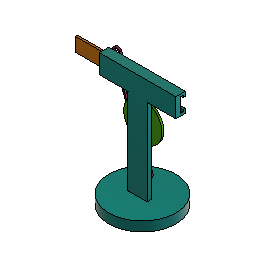
Crank-and-slotted-link-mechanism (Autodesk Fusion 360 design; units mm, degrees)
Autodesk Fusion 360 part; units mm, degrees
sketch "Base" plane through (0, 0, 0) normal (0, 1, 0) x (1, 0, 0) in component "Holder Base"
  circle A0 centre (0, 0) radius 35
  dimension "d1" = 70
  constraint coincident A0.centre origin
  measures "d1" diameter of A0
extrude "Extrude1" add sketch "Base" along normal blind 10 makes body 1 in component "Holder Base"
sketch "Sketch1" plane through (0, 10, 0) normal (0, 1, 0) x (-1, 0, 0)
  circle A0 centre (0, 0) radius 35
sketch "Holder" plane through (0, 10, 0) normal (0, 1, 0) x (-1, 0, 0) in component "Holder"
  line L0 (0, 0) -> (10, 0)
  line L1 (10, 0) -> (10, 5)
  line L2 (10, 5) -> (0, 5)
  line L3 (0, 5) -> (0, 0)
  line L4 (0, 0) -> (-10, 0)
  line L5 (-10, 0) -> (-10, 5)
  line L6 (-10, 5) -> (0, 5)
  line L7 (0, 5) -> (0, 0)
  dimension "d4" = 5
  constraint horizontal L0
  constraint vertical L1
  constraint horizontal L2
  constraint vertical L3
  constraint coincident L0.start L3.end
  constraint horizontal L4
  constraint vertical L5
  constraint horizontal L6
  constraint vertical L7
  measures "d4" distance of L0.start L2.end
sketch "Slot" plane through (0, 10, 0) normal (0, 1, 0) x (-1, 0, 0) in component "Holder Base"
  line L0 (0, 0) -> (10, 0)
  line L1 (10, 0) -> (10, 5)
  line L2 (10, 5) -> (0, 5)
  line L3 (0, 5) -> (0, 0)
  line L4 (0, 0) -> (-10, 0)
  line L5 (-10, 0) -> (-10, 5)
  line L6 (-10, 5) -> (0, 5)
  line L7 (0, 5) -> (0, 0)
  constraint horizontal L0
  constraint vertical L1
  constraint horizontal L2
  constraint vertical L3
  constraint coincident L0.start L3.end
  constraint horizontal L4
  constraint vertical L5
  constraint horizontal L6
  constraint vertical L7
extrude "Extrude2" cut sketch "Slot" against normal blind 15 bodies 1 in component "Holder Base"
extrude "Extrude1'" add sketch "Holder" along normal blind 110 and the other way blind 10 separate body makes body 2 in component "Holder"
sketch "Left arm" plane through (10, 0, 0) normal (1, 0, 0) x (0, 0, -1) in component "Holder"
  line L0 (0, 0) -> (0, 120)
  line L1 (0, 120) -> (-5, 120)
  line L2 (-5, 120) -> (-5, 0)
  line L3 (-5, 0) -> (0, 0)
  line L4 (-5, 120) -> (0, 120)
  line L5 (0, 120) -> (0, 100)
  line L6 (0, 100) -> (-5, 100)
  line L7 (-5, 100) -> (-5, 120)
  constraint horizontal L4
  constraint vertical L5
  constraint horizontal L6
  constraint vertical L7
  constraint coincident L0 L5.end
  constraint coincident L1.end L2.start
sketch "Right arm" plane through (-10, 0, 0) normal (-1, 0, 0) x (0, 0, 1) in component "Holder"
  line L0 (5, 0) -> (5, 120)
  line L1 (5, 120) -> (0, 120)
  line L2 (0, 120) -> (0, 0)
  line L3 (0, 0) -> (5, 0)
  line L4 (0, 120) -> (5, 120)
  line L5 (5, 120) -> (5, 100)
  line L6 (5, 100) -> (0, 100)
  line L7 (0, 100) -> (0, 120)
  constraint horizontal L4
  constraint vertical L5
  constraint horizontal L6
  constraint vertical L7
  constraint coincident L0 L5.end
  constraint coincident L1.end L2.start
extrude "Extrude2'" add sketch "Left arm" along normal blind 30 contours L0 L1 L2 L4 L5 L6 L7 bodies 2 in component "Holder"
extrude "Extrude3" add sketch "Right arm" along normal blind 30 contours L0 L1 L2 L4 L5 L6 L7 bodies 2 in component "Holder"
sketch "Slider holder" plane through (0, 0, 0) normal (0, 0, -1) x (-1, 0, 0) in component "Holder"
  line L0 (10, 0) -> (10, 100)
  line L1 (10, 100) -> (40, 100)
  line L2 (40, 100) -> (40, 120)
  line L3 (40, 120) -> (-40, 120)
  line L4 (-40, 120) -> (-40, 100)
  line L5 (-40, 100) -> (-10, 100)
  line L6 (-10, 100) -> (-10, 0)
  line L7 (-10, 0) -> (10, 0)
  line L8 (-40, 120) -> (40, 120)
  line L9 (40, 120) -> (40, 117.5)
  line L10 (40, 117.5) -> (-40, 117.5)
  line L11 (-40, 117.5) -> (-40, 120)
  line L12 (-40, 100) -> (40, 100)
  line L13 (40, 100) -> (40, 102.5)
  line L14 (40, 102.5) -> (-40, 102.5)
  line L15 (-40, 102.5) -> (-40, 100)
  dimension "d15" = 2.5
  dimension "d16" = 2.5
  constraint horizontal L8
  constraint vertical L9
  constraint horizontal L10
  constraint vertical L11
  constraint coincident L3.end L4.start
  constraint horizontal L12
  constraint vertical L13
  constraint horizontal L14
  constraint vertical L15
  constraint coincident L4.end L5.start
  measures "d15" distance of L3.end L10.end
  measures "d16" distance of L4.end L14.end
extrude "Extrude4" add sketch "Slider holder" along normal blind 5 contours L1 L2 L4 L5 L12 L13 L14 L15 | L2 L3 L4 L8 L9 L10 L11 bodies 2 in component "Holder"
sketch "Slider holder up" plane through (0, 117.5, 0) normal (0, -1, 0) x (1, 0, 0) in component "Holder"
  line L0 (40, 0) -> (-40, 0)
  line L1 (-40, 0) -> (-40, -5)
  line L2 (-40, -5) -> (40, -5)
  line L3 (40, -5) -> (40, 0)
  line L4 (-40, -5) -> (40, -5)
  line L5 (40, -5) -> (40, -2.5)
  line L6 (40, -2.5) -> (-40, -2.5)
  line L7 (-40, -2.5) -> (-40, -5)
  dimension "d19" = 2.5
  constraint horizontal L4
  constraint vertical L5
  constraint horizontal L6
  constraint vertical L7
  constraint coincident L1.end L2.start
  measures "d19" distance of L1.end L6.end
sketch "Slider holder down" plane through (0, 102.5, 0) normal (0, 1, 0) x (-1, 0, 0) in component "Holder"
  line L0 (40, 0) -> (-40, 0)
  line L1 (-40, 0) -> (-40, -5)
  line L2 (-40, -5) -> (40, -5)
  line L3 (40, -5) -> (40, 0)
  line L4 (40, -5) -> (-40, -5)
  line L5 (-40, -5) -> (-40, -2.5)
  line L6 (-40, -2.5) -> (40, -2.5)
  line L7 (40, -2.5) -> (40, -5)
  dimension "d20" = 2.5
  constraint horizontal L4
  constraint vertical L5
  constraint horizontal L6
  constraint vertical L7
  constraint coincident L2.end L3.start
  measures "d20" distance of L2.end L6.end
extrude "Extrude5" add sketch "Slider holder down" along normal blind 2 contours L1 L2 L3 L4 L5 L6 L7 bodies 2 in component "Holder"
extrude "Extrude6" add sketch "Slider holder up" along normal blind 2 contours L1 L2 L3 L4 L5 L6 L7 bodies 2 in component "Holder"
sketch "Slider" plane through (0, 0, 0) normal (0, 0, -1) x (-1, 0, 0) in component "Slider"
  line L0 (40, 117.5) -> (-40, 117.5)
  line L1 (-40, 117.5) -> (-40, 102.5)
  line L2 (-40, 102.5) -> (40, 102.5)
  line L3 (40, 102.5) -> (40, 117.5)
  line L4 (-40, 117.5) -> (40, 117.5)
  line L5 (40, 117.5) -> (40, 102.5)
  line L6 (40, 102.5) -> (-40, 102.5)
  line L7 (-40, 102.5) -> (-40, 117.5)
  constraint horizontal L4
  constraint vertical L5
  constraint horizontal L6
  constraint vertical L7
  constraint coincident L2.end L3.start
  constraint coincident L0.end L1.start
extrude "Extrude1''" add sketch "Slider" along normal blind 2.5 separate body makes body 3 in component "Slider"
move_face "OffsetFaces1" offset -0.3 3 faces at (-13.3333, 117.5, -0.8333) (13.3333, 112.5, -2.5) (13.3333, 102.5, -0.8333) on bodies 3 in component "Slider"
sketch "Pin" plane through (0, 0, -2.2) normal (0, 0, -1) x (-1, 0, 0) in component "Slider"
  line L0 (-40, 102.8) -> (40, 102.8)
  line L1 (40, 102.8) -> (40, 117.2)
  line L2 (40, 117.2) -> (-40, 117.2)
  line L3 (-40, 117.2) -> (-40, 102.8)
  line L4 (40, 117.2) -> (-40, 102.8) construction
  line L5 (-40, 117.2) -> (40, 102.8) construction
  circle A0 centre (0, 110) radius 2.5
  dimension "d32" = 5
  constraint coincident L1.end L2.start
  constraint coincident L0.start L3.end
  constraint coincident L2.end L3.start
  constraint coincident L0.end L1.start
  constraint midpoint L5 A0.centre
  measures "d32" diameter of A0
extrude "Extrude2''" add sketch "Pin" along normal blind 5.1 contours A0 bodies 3 in component "Slider"
move_face "OffsetFaces2" offset -0.7 1 faces at (2.3492, 109.1449, -5.6) on bodies 3 in component "Slider"
sketch "Link holder" plane through (0, 0, 0) normal (0, 0, -1) x (-1, 0, 0) in component "Holder"
  line L0 (10, 100) -> (-10, 100)
  line L1 (-10, 100) -> (-10, 0)
  line L2 (-10, 0) -> (10, 0)
  line L3 (10, 0) -> (10, 100)
  circle A0 centre (0, 25) radius 2.5
  circle A1 centre (0, 25) radius 4.8
  dimension "d37" = 5
  dimension "d41" = 2.3
  measures "d37" diameter of A0
extrude "Extrude7" add sketch "Link holder" along normal blind 7.3 contours A0 bodies 2 in component "Holder"
move_face "OffsetFaces1'" offset -0.3 1 faces at (-2.4876, 24.7511, -2.4333) on bodies 2 in component "Holder"
extrude "Extrude8" add sketch "Link holder" along normal blind 5 contours A1 bodies 2 in component "Holder"
sketch "Link" plane through (0, 0, -7.3) normal (0, 0, -1) x (-1, 0, 0) in component "Link"
  circle A0 centre (0, 25) radius 2.2
  circle A1 centre (0, 25) radius 2.5
  line L0 (30, 110) -> (0, 25)
  line L1 (26.228, 111.3313) -> (-3.772, 26.3313)
  arc A2 (-3.772, 26.3313) -> (3.772, 23.6687) centre (0, 25) ccw
  line L2 (3.772, 23.6687) -> (33.772, 108.6687)
  arc A3 (33.772, 108.6687) -> (26.228, 111.3313) centre (30, 110) ccw
  line L3 (30, 110) -> (0, 25) construction
  line L4 (27.6425, 110.8321) -> (2.681, 40.1078)
  arc A4 (2.681, 40.1078) -> (7.396, 38.4437) centre (5.0385, 39.2757) ccw
  line L5 (7.396, 38.4437) -> (32.3575, 109.168)
  arc A5 (32.3575, 109.168) -> (27.6425, 110.8321) centre (30, 110) ccw
  line L6 (30, 110) -> (5.0385, 39.2757) construction
  line L7 (3.772, 23.6687) -> (37.054, 117.9678)
  arc A6 (37.054, 117.9678) -> (29.5101, 120.6303) centre (33.282, 119.299) ccw
  line L8 (29.5101, 120.6303) -> (-3.772, 26.3313)
  arc A7 (-3.772, 26.3313) -> (3.772, 23.6687) centre (0, 25) ccw
  line L9 (0, 25) -> (33.282, 119.299) construction
  line L10 (7.396, 38.4437) -> (35.6395, 118.467)
  arc A8 (35.6395, 118.467) -> (30.9245, 120.1311) centre (33.282, 119.299) ccw
  line L11 (30.9245, 120.1311) -> (2.681, 40.1078)
  arc A9 (2.681, 40.1078) -> (7.396, 38.4437) centre (5.0385, 39.2757) ccw
  line L12 (5.0385, 39.2757) -> (33.282, 119.299) construction
  dimension "d45" = 0.3
  dimension "d47" = 8
  dimension "d51" = 5
  constraint coincident A0.centre A1.centre
  constraint tangent L1 A2
  constraint tangent A2 L2
  constraint parallel L1 L2
  constraint tangent L2 A3
  constraint tangent L1 A3
  constraint parallel L0 L3
  constraint tangent L4 A4
  constraint tangent A4 L5
  constraint parallel L4 L5
  constraint tangent L5 A5
  constraint tangent L4 A5
  constraint parallel L0 L6
  constraint coincident L0.start A3.centre
  constraint tangent L7 A6
  constraint tangent A6 L8
  constraint parallel L7 L8
  constraint tangent L8 A7
  constraint tangent L7 A7
  constraint parallel L0 L9
  constraint tangent L10 A8
  constraint tangent A8 L11
  constraint parallel L10 L11
  constraint tangent L11 A9
  constraint tangent L10 A9
  constraint coincident A6.centre L9.end
  constraint parallel L9 L12
  constraint coincident A4.centre L6.end
  measures "d47" diameter of A2
  measures "d51" diameter of A4
sketch "Crank holder" plane through (0, 0, 0) normal (0, 0, -1) x (-1, 0, 0) in component "Holder"
  line L0 (10, 100) -> (-10, 100)
  line L1 (-10, 100) -> (-10, 0)
  line L2 (-10, 0) -> (10, 0)
  line L3 (10, 0) -> (10, 100)
  circle A0 centre (0, 25) radius 4.8
  circle A1 centre (0, 75) radius 2.5
  dimension "d48" = 5
  measures "d48" diameter of A1
extrude "Extrude9" add sketch "Crank holder" along normal blind 2.5 contours A1 bodies 2 in component "Holder"
extrude "Extrude1'''" add sketch "Link" against normal blind 2 separate body contours L1 A2 L2 A3 L4 A4 L5 L7 L8 A7 L10 L11 A9 | A3 L7 A6 L8 L10 A8 L11 makes body 4 in component "Link"
sketch "Crank" plane through (0, 0, -2.5) normal (0, 0, -1) x (-1, 0, 0) in component "Crank"
  circle A0 centre (0, 75) radius 2.5
  line L0 (0, 75) -> (19.6175, 68.0762) construction
  line L1 (3.772, 23.6687) -> (37.054, 117.9678)
  circle A1 centre (0, 75) radius 20
  line L2 (13.3352, 70.2935) -> (18.05, 68.6294)
  circle A2 centre (15.6926, 69.4614) radius 2.5
  dimension "d58" = 40
  dimension "d62" = 5
  constraint coincident A0.centre L0.start
  constraint perpendicular L0 L1
  constraint coincident L0 L2.start
  constraint coincident L0 L2.end
  constraint midpoint L2 A2.centre
  measures "d58" diameter of A1
  measures "d62" diameter of A2
extrude "Extrude1''''" add sketch "Crank" against normal blind 2 separate body contours A1 | L2 A2 | L2 A2 makes body 5 in component "Crank"
move_face "OffsetFaces2'" offset -0.3 1 faces at (-2.3492, 74.145, -1.6667) on bodies 2 in component "Holder"
extrude "Extrude2'''" add sketch "Crank" along normal blind 4.8 contours L2 A2 | L2 A2 bodies 5 in component "Crank"
move_face "OffsetFaces1''" offset -0.7 1 faces at (-13.3434, 70.3165, -5.7) on bodies 5 in component "Crank"
component "Holder Base" placed x (1, 0, 0) y (0, 1, 0) z (0, 0, 1) at (0, 0, 0)
component "Holder" placed x (1, 0, 0) y (0, 1, 0) z (0, 0, 1) at (0, 0, 0)
component "Slider" placed x (1, 0, 0) y (0, 1, 0) z (0, 0, 1) at (-30, 0, 0)
component "Link" placed x (0.99997, -0.007766, 0) y (0.007766, 0.99997, 0) z (0, 0, 1) at (-0.1941, 0.0008, 0)
component "Crank" placed x (0.996917, -0.078459, 0) y (0.078459, 0.996917, 0) z (0, 0, 1) at (-5.8844, 0.2312, 0)
named bodies: "Holder Base", "Holder", "Slider", "Crank"
